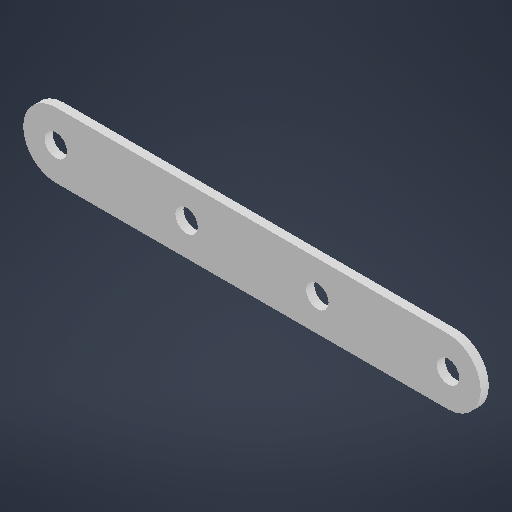
# Autodesk Inventor part: 2ndpreroller
Saved by Autodesk Inventor 2025.2 (Build 292293000, 293)
## iProperties
Created: 2025-01-15
Part Number: 2ndpreroller
Material: Polycarbonate, Clear
Document SubType Name: Sheet Metal
Designer: Jahan
Density: 1.2 g/cm^3
Appearance: Polycarbonate - Clear
Flat Pattern Width: 1.27 cm
Flat Pattern Length: 8.89 cm
Flat Pattern Area: 11.2903 cm^2
Sheet Metal Rule: Default
Sheet Metal Width: 0.500 in
Sheet Metal Length: 3.500 in
Sheet Metal Area: 1.750 in^2
Author: Jahan
Autodesk Inventor part; units mm, degrees
ref_plane "YZ Plane" through (0, 0, 0) normal (1, 0, 0) x (0, 1, 0)
ref_plane "XZ Plane" through (0, 0, 0) normal (0, 1, 0) x (-1, 0, 0)
ref_plane "XY Plane" through (0, 0, 0) normal (0, 0, 1) x (1, 0, 0)
sketch "Sketch1" plane through (0, 0, 0) normal (0, 0, 1) x (1, 0, 0)
  circle A0 centre (0, 0) radius 2.1844
  circle A1 centre (76.2, 0) radius 2.1844
  circle A2 centre (25.4, 0) radius 2.1844
  circle A3 centre (50.8, 0) radius 2.1844
  line L0 (0, -6.35) -> (76.2, -6.35)
  arc A4 (76.2, -6.35) -> (76.2, 6.35) centre (76.2, 0) ccw
  line L1 (76.2, 6.35) -> (0, 6.35)
  arc A5 (0, 6.35) -> (0, -6.35) centre (0, 0) ccw
  dimension "d0" = 4.3688
  dimension "d6" = 4.3688
  dimension "d12" = 4.3688
  dimension "d13" = 25.4
  dimension "d14" = 76.2
  dimension "d15" = 4.3688
  dimension "d16" = 25.4
  dimension "d17" = 76.2
  dimension "d20" = 76.2
  constraints: 6 centre point, 4 end point, 4 point on circle, 3 coincident, 2 horizontal
  measures "d0" diameter of A0
  measures "d6" diameter of A1
  measures "d12" diameter of A2
  measures "d13" distance of A2.centre point (0, 0)
  measures "d14" distance of A1.centre point (0, 0)
  measures "d15" diameter of A3
  measures "d16" distance of A1.centre A3.centre
  measures "d17" distance of L0.start L0.end
  measures "d20" distance of L1.start L1.end
extrude "Extrusion2" add sketch "Sketch1" along normal blind 1.5875
body "Solid2"
